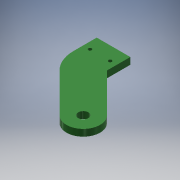
# Autodesk Inventor part: Cross Arms
Saved by Autodesk Inventor 2017 (Build 210142000, 142)
## iProperties
Created: 2017-01-12
Part Number: Cross Arms
Material: Generic
Document SubType Name: Modeling
Designer: Ben
Density: 1 g/cm^3
Appearance: Smooth - Dark Forest Green
Author: Ben
Autodesk Inventor part; units mm, degrees
ref_plane "YZ Plane" through (0, 0, 0) normal (1, 0, 0) x (0, 1, 0)
ref_plane "XZ Plane" through (0, 0, 0) normal (0, 1, 0) x (-1, 0, 0)
ref_plane "XY Plane" through (0, 0, 0) normal (0, 0, 1) x (1, 0, 0)
sketch "Sketch1" plane through (0, 0, 0) normal (0, 1, 0) x (-1, 0, 0)
  circle A0 centre (0, 0) radius 4.7625
  line L0 (0, -228.6) -> (0, 0) construction
  line L1 (15.875, -228.6) -> (0, -228.6) construction
  circle A1 centre (15.875, -228.6) radius 7.9375
  line L2 (25.4, -47.8506) -> (25.4, -212.725)
  line L3 (57.15, -47.8506) -> (57.15, -212.725)
  line L4 (25.4, -212.725) -> (15.875, -212.725)
  arc A2 (15.875, -212.725) -> (15.875, -244.475) centre (15.875, -228.6) ccw
  line L5 (15.875, -244.475) -> (25.4, -244.475)
  arc A3 (25.4, -244.475) -> (57.15, -212.725) centre (25.4, -212.725) ccw
  line L6 (57.15, -130.2878) -> (25.4, -130.2878) construction
  arc A4 (11.2253, 11.2253) -> (-11.2253, -11.2253) centre (0, 0) ccw
  line L7 (-11.2253, -11.2253) -> (25.4, -47.8506)
  arc A5 (57.15, -47.8506) -> (47.8506, -25.4) centre (25.4, -47.8506) ccw
  line L8 (47.8506, -25.4) -> (11.2253, 11.2253)
  line L9 (41.275, -130.2878) -> (41.275, -240.2213) construction
  line L10 (41.275, -130.2878) -> (41.275, -18.8244) construction
  dimension "d0" = 9.525
  dimension "d2" = 228.6
  dimension "d7" = 15.875
  dimension "d17" = 31.75
  dimension "d18" = 45
  dimension "d19" = 25.4
  dimension "d20" = 25.4
  constraints: 23 end point, 9 point on circle, 8 tangent, 6 centre point, 5 vertical, 4 coincident, 3 horizontal, 3 midpoint, 1 equal radius, 1 parallel, 1 perpendicular, 1 point on line
  measures "d0" diameter of A0
  measures "d2" distance of point (0, 0) L0.start
  measures "d7" diameter of A1
  measures "d17" diameter of A4
  measures "d18" angle of L2 L7
  measures "d19" distance from line of L1.start L9
  measures "d20" distance between parallel lines of L0 L2
extrude "Extrusion1" add sketch "Sketch1" along normal blind 6.35
sketch "Sketch2" plane through (0, 6.35, 0) normal (0, 1, 0) x (1, 0, 0)
  line L0 (-69.0057, 276.0917) -> (22.485, 276.0917)
  line L1 (22.485, 276.0917) -> (22.485, 69.85)
  line L2 (22.485, 69.85) -> (-69.0057, 69.85)
  line L3 (-69.0057, 69.85) -> (-69.0057, 276.0917)
  point P0 (0, 0)
  dimension "d21" = 69.85
  constraints: 8 end point, 2 parallel, 1 horizontal, 1 perpendicular
  measures "d21" distance from line of point (0, 0) L2
extrude "Extrusion2" cut sketch "Sketch2" against normal through all
sketch "Sketch3" plane through (0, 6.35, 0) normal (0, 1, 0) x (1, 0, 0)
  line L0 (-25.4, 47.8506) -> (-25.4, 69.85) construction
  line L1 (-25.4, 47.8506) -> (-25.4, 69.85) construction
  line L2 (-25.4, 57.15) -> (-57.15, 57.15) construction
  line L3 (-25.4, 69.85) -> (-57.15, 69.85) construction
  line L4 (-41.275, 69.85) -> (-41.275, 57.15) construction
  circle A0 centre (-50.8, 57.15) radius 1.5875
  circle A1 centre (-31.75, 57.15) radius 1.5875
  point P0 (0, 0)
  dimension "d24" = 12.7
  dimension "d26" = 3.175
  dimension "d27" = 19.05
  constraints: 4 end point, 3 point on line, 2 centre point, 2 midpoint, 1 equal radius, 1 horizontal, 1 vertical, 1 other
  measures "d24" distance between parallel lines of L3 L2
  measures "d26" diameter of A1
  measures "d27" distance of A0.centre A1.centre
extrude "Extrusion3" cut sketch "Sketch3" against normal through all
body "Solid1"
